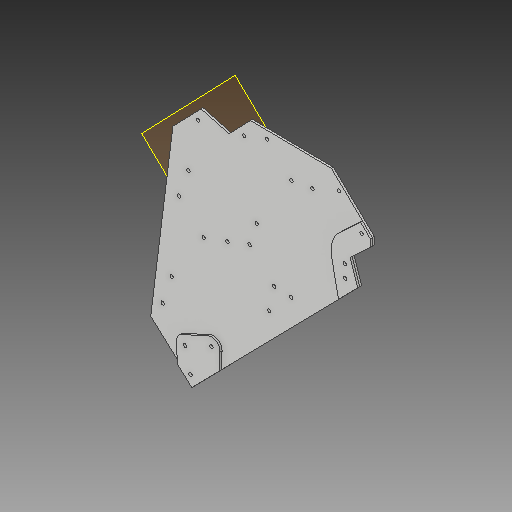
# Autodesk Inventor part: PlateRight
Saved by Autodesk Inventor 2019.2 (Build 232265000, 265)
## iProperties
Created: 2018-09-29
Part Number: PlateRight
Material: Generic
Document SubType Name: Modeling
Designer: eroldan
Density: 1 g/cm^3
Appearance: Default
Author: eroldan
Autodesk Inventor part; units mm, degrees
ref_plane "YZ Plane" through (0, 0, 0) normal (1, 0, 0) x (0, 1, 0)
ref_plane "XZ Plane" through (0, 0, 0) normal (0, 1, 0) x (-1, 0, 0)
ref_plane "XY Plane" through (0, 0, 0) normal (0, 0, 1) x (1, 0, 0)
ref_plane "Work Plane1" through (78.9702, 307.1183, 35) normal (0, 0, 1) x (0.6934, 0.7205, 0)
sketch "Sketch1" plane through (78.9702, 307.1183, 35) normal (0, 0, 1) x (0.6934, 0.7205, 0)
  line L0 (-245.8377, -151.2647) -> (102.2371, -154.4014)
  line L1 (102.2371, -154.4014) -> (118.2728, -123.5)
  line L2 (118.2728, -123.5) -> (166.8824, -126)
  line L3 (166.8824, -126) -> (166.8824, -34.5067)
  line L4 (166.8824, -34.5067) -> (85.4836, 52.2409)
  line L5 (-40.0118, 89.6338) -> (-248.2508, -65.6521)
  line L6 (-248.2508, -65.6521) -> (-245.8377, -151.2647)
  circle A0 centre (61.694, 42) radius 2.5 projected
  circle A1 centre (-56.306, 42) radius 2.5 projected
  circle A2 centre (94, 26.8002) radius 2.5 projected
  circle A3 centre (94, -23.1998) radius 2.5 projected
  circle A4 centre (118.7923, -42) radius 2.5 projected
  circle A5 centre (158.2014, -58.3927) radius 2.5 projected
  circle A6 centre (158.2014, -108.3927) radius 2.5 projected
  circle A7 centre (104.7371, -126) radius 2.5 projected
  circle A8 centre (-13.2629, -126) radius 2.5 projected
  circle A9 centre (-29.7986, -106.987) radius 2.5 projected
  circle A10 centre (-29.7986, -56.987) radius 2.5 projected
  circle A11 centre (0.7923, -42) radius 2.5 projected
  circle A12 centre (-61.3802, -42) radius 2.5 projected
  circle A13 centre (-94, -25.2342) radius 2.5 projected
  circle A14 centre (-94, 24.7658) radius 2.5 projected
  circle A15 centre (-217.7986, -110.5404) radius 2.5 projected
  circle A16 centre (-177.91, -126) radius 2.5 projected
  circle A17 centre (-217.7986, -60.5404) radius 2.5 projected
  circle A18 centre (-179.3802, -42) radius 2.5 projected
  circle A19 centre (-59.91, -126) radius 2.5 projected
  line L7 (85.4836, 52.2409) -> (40.182, 52.2409)
  line L8 (40.182, 52.2409) -> (19.661, 89.6338)
  line L9 (19.661, 89.6338) -> (-40.0118, 89.6338)
  circle A20 centre (4.6388, 81.3897) radius 2.5
  circle A21 centre (-235.861, -138.9507) radius 2.5
  circle A22 centre (91.5, -138.9507) radius 2.5
  point P0 (-276.0496, -156.0595)
  dimension "d5" = 5
  dimension "d6" = 5
  dimension "d7" = 5
  constraints: 20 end point, 3 centre point, 1 parallel
  measures "d5" diameter of A20
  measures "d6" diameter of A21
  measures "d7" diameter of A22
extrude "Extrusion1" add sketch "Sketch1" along normal blind 3
chamfer "Chamfer1" distance 8 angle 45 1 edges at (285.4768, 339.9931, 36.5)
sketch "Sketch2" plane through (78.9702, 307.1183, 38) normal (0, 0, 1) x (0.7205, -0.6934, 0)
  line L0 (65.6521, -248.2508) -> (151.2647, -245.8377) construction
  line L1 (151.2647, -245.8377) -> (154.4014, 102.2371) construction
  line L2 (151.2647, -245.8377) -> (122.4128, -246.6509)
  line L3 (122.4128, -246.6509) -> (101.8549, -226.7882)
  line L4 (135.2303, -169.4804) -> (151.7873, -187.8491)
  line L5 (151.7873, -187.8491) -> (151.2647, -245.8377)
  circle A0 centre (138.9507, -235.861) radius 2.5 projected
  circle A1 centre (110.5404, -217.7986) radius 2.5 projected
  circle A2 centre (126, -177.91) radius 2.5 projected
  arc A3 (98.8852, -213.2814) -> (101.8549, -226.7882) centre (110.5404, -217.7986) ccw
  arc A4 (135.2848, -169.5409) -> (114.3448, -173.3928) centre (126, -177.91) ccw
  line L6 (114.3448, -173.3928) -> (98.8852, -213.2814)
  point P0 (156.0595, -276.0496)
  dimension "d8" = 10
  dimension "d9" = 10
  constraints: 10 end point, 4 point on circle, 3 point on line, 3 tangent, 2 centre point, 1 collinear
  measures "d8" radial gap between concentric circles of A1 A3
  measures "d9" radial gap between concentric circles of A2 A4
extrude "Extrusion2" add sketch "Sketch2" along normal blind 3 separate body
sketch "Sketch3" plane through (78.9702, 307.1183, 38) normal (0, 0, 1) x (0.7205, -0.6934, 0)
  line L0 (154.4014, 102.2371) -> (123.5, 118.2728) projected
  line L1 (151.2647, -245.8377) -> (154.4014, 102.2371) projected
  line L2 (154.0397, 62.0952) -> (94.5868, 102.7761)
  line L3 (118, 166.8824) -> (34.5067, 166.8824) construction
  line L4 (125.5891, 158.8929) -> (118, 166.8824) projected
  line L5 (123.5, 118.2728) -> (125.5891, 158.8929) projected
  line L6 (94.5868, 102.7761) -> (97.8838, 166.8824)
  line L7 (118, 166.8824) -> (97.8838, 166.8824)
  circle A0 centre (108.3927, 158.2014) radius 2.5 projected
  circle A1 centre (126, 104.7371) radius 2.5 projected
  circle A2 centre (138.9507, 91.5) radius 2.5 projected
  point P0 (156.0595, -276.0496)
  constraints: 6 end point, 2 point on line, 1 collinear
extrude "Extrusion3" add sketch "Sketch3" along normal blind 3 separate body
fillet "Fillet1" radius 38.75 1 edges at (218.3902, 315.5845, 39.5)
